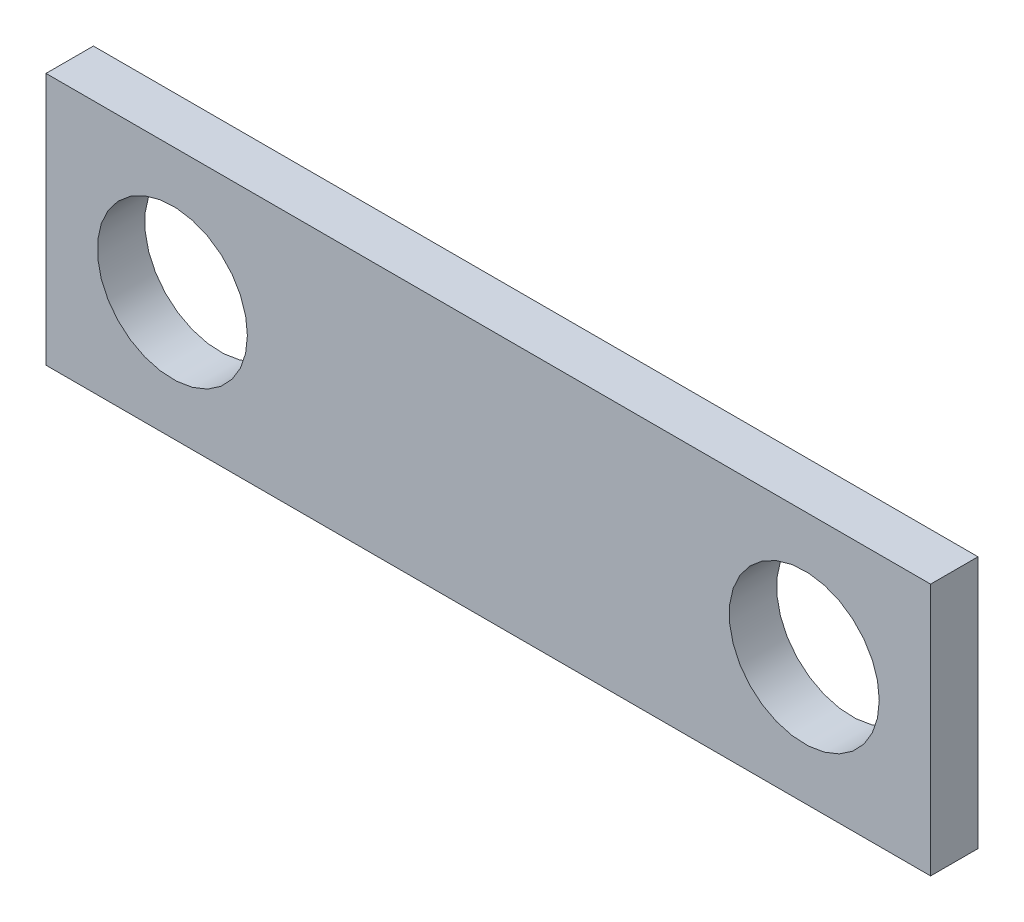
# Autodesk Inventor part: Connector
Saved by Autodesk Inventor 2016 (Build 200138000, 138)
## iProperties
Created: 2017-03-04
Part Number: Connector
Material: Generic
Document SubType Name: Modeling
Designer: Owner
Density: 1 g/cm^3
Appearance: Default
Author: Owner
Autodesk Inventor part; units mm, degrees
ref_plane "YZ Plane" through (0, 0, 0) normal (1, 0, 0) x (0, 1, 0)
ref_plane "XZ Plane" through (0, 0, 0) normal (0, 1, 0) x (-1, 0, 0)
ref_plane "XY Plane" through (0, 0, 0) normal (0, 0, 1) x (1, 0, 0)
sketch "Sketch2" plane through (0, 0, 0) normal (0, 0, 1) x (1, 0, 0)
  circle A0 centre (7.019, 0.1365) radius 2.125 projected
  circle A1 centre (7.019, 0.1365) radius 2.375
  line L0 (7.019, 0.1365) -> (7.019, 4.1365)
  line L1 (7.019, 4.1365) -> (3.019, 4.1365)
  line L2 (3.019, 4.1365) -> (31.019, 4.1365)
  line L3 (31.019, 4.1365) -> (31.019, -3.8635)
  line L4 (31.019, -3.8635) -> (3.019, -3.8635)
  line L5 (3.019, -3.8635) -> (3.019, 4.1365)
  line L6 (17.019, 4.1365) -> (17.019, 2)
  circle A2 centre (27.019, 0.1365) radius 2.375
  point P0 (0, 0)
  dimension "d0" = 4.75
  dimension "d1" = 4
  dimension "d2" = 4
  dimension "d3" = 28
  dimension "d4" = 8
  constraints: 14 end point, 2 centre point, 2 parallel, 2 perpendicular, 2 vertical, 1 coincident, 1 horizontal, 1 midpoint, 1 symmetric about line, 1 other
  measures "d0" diameter of A1
  measures "d1" distance of L0.start L0.end
  measures "d2" distance of L0.end L1.end
  measures "d3" distance of L1.end L2.end
  measures "d4" distance of L4.end L1.end
extrude "Extrusion1" add sketch "Sketch2" along normal blind 1.5 contours L2 L3 L4 L5 L1
body "Solid1"
